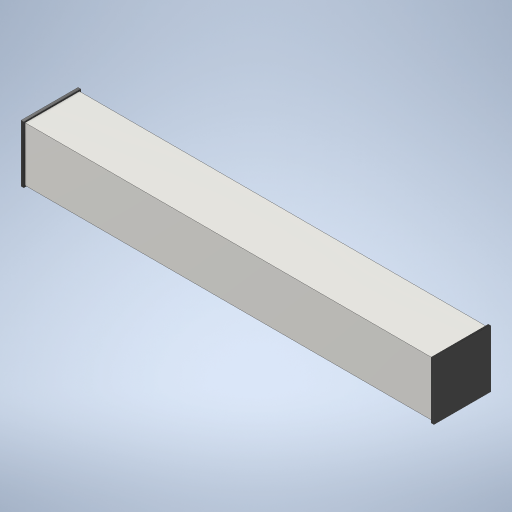
# Autodesk Inventor part: InoxLienKet
Saved by Autodesk Inventor 2023 (Build 270158000, 158)
## iProperties
Created: 2025-03-24
Part Number: InoxLienKet
Material: Generic
Document SubType Name: Modeling
Designer: huyqu
Density: 1 g/cm^3
Appearance: Default
Author: huyqu
Autodesk Inventor part; units mm, degrees
ref_plane "YZ Plane" through (0, 0, 0) normal (1, 0, 0) x (0, 1, 0)
ref_plane "XZ Plane" through (0, 0, 0) normal (0, 1, 0) x (-1, 0, 0)
ref_plane "XY Plane" through (0, 0, 0) normal (0, 0, 1) x (1, 0, 0)
sketch "Sketch1" plane through (0, 0, 0) normal (0, 0, 1) x (1, 0, 0)
  line L0 (0, 0) -> (300, 0)
  line L1 (0, 0) -> (0, -40)
  line L2 (0, -40) -> (300, -40)
  line L3 (300, -40) -> (300, 0)
  dimension "d0" = 300
  dimension "d1" = 40
  constraints: 8 end point, 2 horizontal, 1 perpendicular, 1 vertical
  measures "d0" distance of L0.start L0.end
  measures "d1" distance of L0.start L1.end
extrude "Extrusion1" add sketch "Sketch1" along normal blind 40
sketch "Sketch2" plane through (300, -40, 0) normal (1, 0, 0) x (0, 0, -1)
  line L0 (1, 41) -> (-41, 41)
  line L1 (0, 40) -> (-40, 40) projected
  line L2 (1, 41) -> (1, -1)
  line L3 (-41, 41) -> (-41, -1)
  line L4 (-41, -1) -> (1, -1)
  line L5 (0, 0) -> (0, 40) projected
  dimension "d4" = 1
  dimension "d5" = 42
  dimension "d6" = 42
  dimension "d7" = 1
  constraints: 8 end point, 2 vertical, 1 horizontal, 1 perpendicular
  measures "d4" distance between parallel lines of L1 L0
  measures "d5" distance of L0.start L0.end
  measures "d6" distance of L0.start L2.end
  measures "d7" distance between parallel lines of L5 L2
extrude "Extrusion2" add sketch "Sketch2" along normal blind 2
sketch "Sketch3" plane through (0, -40, 0) normal (-1, 0, 0) x (0, 0, 1)
  line L0 (-1, 41) -> (41, 41) projected
  line L1 (41, 41) -> (41, -1) projected
  line L2 (41, 41) -> (41, -1)
  line L3 (41, -1) -> (-1, -1) projected
  line L4 (41, -1) -> (-1, -1)
  line L5 (-1, -1) -> (-1, 41) projected
  line L6 (-1, -1) -> (-1, 41)
  line L7 (-1, 41) -> (41, 41)
  point P0 (0, 40)
  constraints: 8 end point, 2 collinear, 2 perpendicular
extrude "Extrusion3" add sketch "Sketch3" along normal blind 2
body "Solid1"
